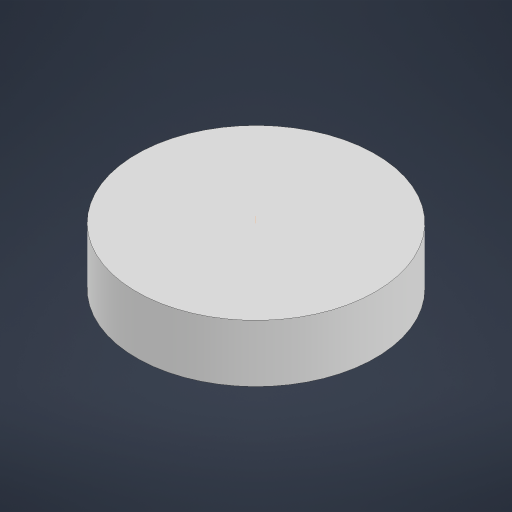
# Autodesk Inventor part: Button_adapter
Saved by Autodesk Inventor 2023 (Build 270158030, 158C)
## iProperties
Created: 2022-06-02
Part Number: Button_adapter
Material: Generic
Document SubType Name: Modeling
Designer: Simon
Density: 1 g/cm^3
Appearance: Default
Author: Simon
Autodesk Inventor part; units mm, degrees
ref_plane "YZ Plane" through (0, 0, 0) normal (1, 0, 0) x (0, 1, 0)
ref_plane "XZ Plane" through (0, 0, 0) normal (0, 1, 0) x (-1, 0, 0)
ref_plane "XY Plane" through (0, 0, 0) normal (0, 0, 1) x (1, 0, 0)
sketch "Sketch1" plane through (0, 0, 0) normal (0, 1, 0) x (-1, 0, 0)
  circle A0 centre (0, 0) radius 5.85
  circle A1 centre (0, 0) radius 15
  dimension "d0" = 11.7
  dimension "d1" = 30
  constraints: 2 centre point, 2 coincident
  measures "d0" diameter of A0
  measures "d1" diameter of A1
extrude "Extrusion1" add sketch "Sketch1" along normal blind 4.2
sketch "Sketch2" plane through (0, 4.2, 0) normal (0, 1, 0) x (1, 0, 0)
  circle A0 centre (0, 0) radius 15 projected
extrude "Extrusion2" add sketch "Sketch2" along normal blind 3
shell "Shell1" thickness 1.5 removed faces 1 at (-11.748, 0, -1.6632)
sketch "Sketch3" plane through (0, 0, 0) normal (1, 0, 0) x (0, 1, 0)
  line L0 (5.7, -13.5) -> (5.7, 13.5) projected
  line L1 (5.7, 7.35) -> (0, 7.35) projected
  arc A0 (5.7, 13.5) -> (5.7, 7.35) centre (8.2582, 10.425) ccw
  line L2 (-1.6516, 0) -> (9.9098, 0) projected
  point P0 (0, 0)
  dimension "d7" = 4
  constraints: 2 point on circle, 1 centre point, 1 point on line
  measures "d7" radius of A0
revolve "Revolution1" add sketch "Sketch3" angle 360 about axis through (0, -10, 0) along (0, 1, 0)
fillet "Fillet1" radius 1.5 2 edges at (5.1969, 5.7, -5.1976) (-5.1969, 5.7, 5.1976)
body "Solid1"
